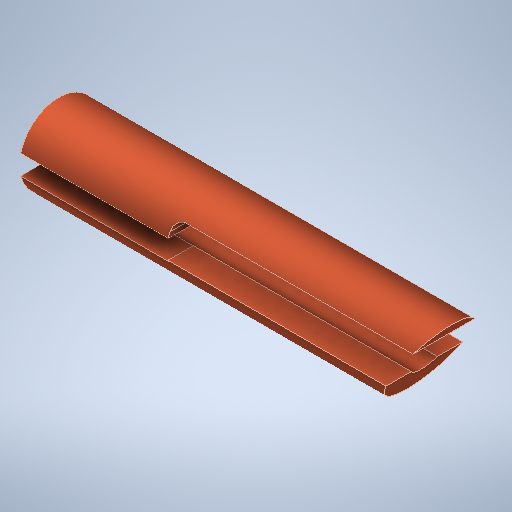
# Autodesk Inventor part: Main_tip_coupler
Saved by Autodesk Inventor 2026.2 (Build 302298010, 298A)
## iProperties
Created: 2026-05-11
Part Number: Main_tip_coupler
Material: Generic
Document SubType Name: Modeling
Designer: piete
Density: 1 g/cm^3
Appearance: Copper - Satin
Author: piete
Autodesk Inventor part; units mm, degrees
ref_plane "YZ Plane" through (0, 0, 0) normal (1, 0, 0) x (0, 1, 0)
ref_plane "XZ Plane" through (0, 0, 0) normal (0, 1, 0) x (-1, 0, 0)
ref_plane "XY Plane" through (0, 0, 0) normal (0, 0, 1) x (1, 0, 0)
sketch "Sketch1" plane through (0, 0, 0) normal (1, 0, 0) x (0, 1, 0)
  circle A0 centre (0, 0) radius 4
  dimension "d0" = 8
  constraints: 1 centre point, 1 coincident
  measures "d0" diameter of A0
extrude "Extrusion1" add sketch "Sketch1" along normal blind 40
sketch "Sketch2" plane through (40, 0, 0) normal (1, 0, 0) x (0, 0, -1)
  line L0 (-4, 2.5) -> (4, 2.5)
  line L1 (4, 2.5) -> (4, -0.9)
  line L2 (4, -0.9) -> (-4, -0.9)
  line L3 (-4, -0.9) -> (-4, 2.5)
  point P0 (0, 0)
  dimension "d3" = 8
  dimension "d4" = 3.4
  dimension "d5" = 2.5
  dimension "d6" = 4
  constraints: 8 end point, 2 parallel, 1 horizontal, 1 perpendicular
  measures "d3" distance of L1.end L2.end
  measures "d4" distance of L0.end L1.end
  measures "d5" distance from line of point (0, 0) L0
  measures "d6" distance from line of point (0, 0) L1
extrude "Extrusion2" cut sketch "Sketch2" against normal blind 25
sketch "Sketch3" plane through (0, 0, 0) normal (-1, 0, 0) x (0, 0, 1)
  circle A0 centre (0, 0) radius 1.6
  dimension "d9" = 3.2
  constraints: 1 centre point, 1 coincident
  measures "d9" diameter of A0
extrude "Extrusion3" cut sketch "Sketch3" against normal through all
sketch "Sketch4" plane through (0, 0, 0) normal (0, 0, 1) x (1, 0, 0)
  line L0 (40, 2.5) -> (40, 4) projected
  line L1 (40, 4) -> (35.3812, -4)
  line L2 (0, -4) -> (40, -4) projected
  line L3 (40, 4) -> (49.2376, 4) construction
  line L4 (35.3812, -4) -> (40, -4)
  line L5 (40, 4) -> (40, -4)
  point P0 (0, 0)
  dimension "d12" = 120
  constraints: 8 end point, 2 point on line, 1 equal length, 1 horizontal, 1 perpendicular
  measures "d12" angle of L1 L3
extrude "Extrusion4" cut sketch "Sketch4" along normal through all both and the other way through all
sketch "Sketch6" plane through (0, 0, 0) normal (-1, 0, 0) x (0, 0, 1)
  line L0 (4, 1) -> (1.2, 1)
  line L1 (1.2, 1) -> (1.2, -1)
  line L2 (1.2, -1) -> (4, -1)
  line L3 (4, -1) -> (4, 1)
  point P0 (0, 0)
  dimension "d23" = 2
  dimension "d24" = 4
  dimension "d25" = 1
  dimension "d27" = 1.2
  constraints: 8 end point, 2 parallel, 1 horizontal, 1 perpendicular
  measures "d23" distance of L1.end L0.end
  measures "d24" distance from line of point (0, 0) L3
  measures "d25" distance from line of point (0, 0) L0
  measures "d27" distance from line of point (0, 0) L1
extrude "Extrusion6" cut sketch "Sketch6" against normal up to surface (15 mm away)
fillet "Fillet1" radius 1 1 edges at (15, 2.5, 0)
fillet "Fillet2" radius 1 1 edges at (15, -0.9, -2.6102)
equation "\"d6\" = 0.5 * d3"
equation "\"d25\" = 0.5 * d23"
body "Solid1"
